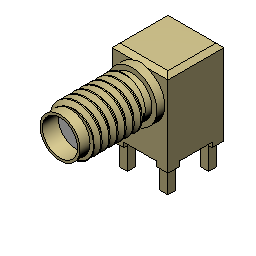
L-KLS1-SMA006 (Autodesk Fusion 360 design; units mm, degrees)
Autodesk Fusion 360 part; units mm, degrees
sketch "Sketch1" plane through (0, 0, 0) normal (0, 0, 1) x (1, 0, 0)
  circle A0 centre (0, 0) radius 0.65
  circle A1 centre (2.54, 2.54) radius 0.8
  circle A2 centre (-2.54, 2.54) radius 0.8
  circle A3 centre (-2.54, -2.54) radius 0.8
  circle A4 centre (2.54, -2.54) radius 0.8
  line L0 (3.04, 2.04) -> (2.04, 2.04)
  line L1 (2.04, 2.04) -> (2.04, 3.04)
  line L2 (2.04, 3.04) -> (3.04, 3.04)
  line L3 (3.04, 3.04) -> (3.04, 2.04)
  line L4 (3.04, 2.04) -> (2.04, 3.04) construction
  line L5 (2.04, 2.04) -> (3.04, 3.04) construction
  line L6 (-2.04, 2.04) -> (-3.04, 2.04)
  line L7 (-3.04, 2.04) -> (-3.04, 3.04)
  line L8 (-3.04, 3.04) -> (-2.04, 3.04)
  line L9 (-2.04, 3.04) -> (-2.04, 2.04)
  line L10 (-2.04, 2.04) -> (-3.04, 3.04) construction
  line L11 (-3.04, 2.04) -> (-2.04, 3.04) construction
  line L12 (-2.04, -2.04) -> (-3.04, -2.04)
  line L13 (-3.04, -2.04) -> (-3.04, -3.04)
  line L14 (-3.04, -3.04) -> (-2.04, -3.04)
  line L15 (-2.04, -3.04) -> (-2.04, -2.04)
  line L16 (-2.04, -2.04) -> (-3.04, -3.04) construction
  line L17 (-3.04, -2.04) -> (-2.04, -3.04) construction
  line L18 (3.04, -3.04) -> (2.04, -3.04)
  line L19 (2.04, -3.04) -> (2.04, -2.04)
  line L20 (2.04, -2.04) -> (3.04, -2.04)
  line L21 (3.04, -2.04) -> (3.04, -3.04)
  line L22 (3.04, -3.04) -> (2.04, -2.04) construction
  line L23 (2.04, -3.04) -> (3.04, -2.04) construction
  line L24 (3.5, 3.5) -> (3.5, -3.5)
  line L25 (-3.5, 3.5) -> (3.5, 3.5)
  line L26 (-3.5, -3.5) -> (-3.5, 3.5)
  line L27 (3.5, -3.5) -> (-3.5, -3.5)
  point P0 (2.54, 2.54)
  point P1 (2.54, 2.54)
  point P2 (-2.54, 2.54)
  point P3 (-2.54, -2.54)
  point P4 (2.54, -2.54)
  dimension "d1" = 1.3
  dimension "d2" = 1
  dimension "d3" = 1
  dimension "d4" = 1
  dimension "d5" = 1
  dimension "d6" = 1
  dimension "d7" = 1
  dimension "d8" = 1
  dimension "d9" = 1
  constraint coincident A0.centre origin
  constraint horizontal L0
  constraint perpendicular L0 L1
  constraint parallel L0 L2
  constraint parallel L1 L3
  constraint coincident L4 P1
  constraint coincident L5 P1
  constraint coincident P1 P0
  constraint horizontal L6
  constraint perpendicular L6 L7
  constraint parallel L6 L8
  constraint parallel L7 L9
  constraint coincident L10 P2
  constraint coincident L11 P2
  constraint coincident P2 A2.centre
  constraint horizontal L12
  constraint perpendicular L12 L13
  constraint parallel L12 L14
  constraint parallel L13 L15
  constraint coincident L16 P3
  constraint coincident L17 P3
  constraint coincident P3 A3.centre
  constraint horizontal L18
  constraint perpendicular L18 L19
  constraint parallel L18 L20
  constraint parallel L19 L21
  constraint coincident L22 P4
  constraint coincident L23 P4
  constraint coincident P4 A4.centre
  measures "d1" diameter of A0
  measures "d2" distance of L1.end L2.end
  measures "d3" distance of L0.end L1.end
  measures "d4" distance of L7.end L8.end
  measures "d5" distance of L6.end L7.end
  measures "d6" distance of L13.end L14.end
  measures "d7" distance of L12.end L13.end
  measures "d8" distance of L19.end L20.end
  measures "d9" distance of L18.end L19.end
extrude "Extrude1" add sketch "Sketch1" along normal blind 10.6 contours A0 | A1 | A2 | A3 | A4 | L0 L1 L2 L3 | L6 L7 L8 L9 | L12 L13 L14 L15 | L18 L19 L20 L21 | L24 L25 L26 L27
sketch "Sketch2" plane through (0, 0, 0) normal (0, 0, -1) x (1, 0, 0)
  line L0 (3.5, -3.5) -> (3.5, 3.5)
  line L1 (3.5, 3.5) -> (-3.5, 3.5)
  line L2 (-3.5, 3.5) -> (-3.5, -3.5)
  line L3 (-3.5, -3.5) -> (3.5, -3.5)
  circle A0 centre (2.54, 2.54) radius 0.8
  circle A1 centre (-2.54, 2.54) radius 0.8
  circle A2 centre (0, 0) radius 0.8
  circle A3 centre (-2.54, -2.54) radius 0.8
  circle A4 centre (2.54, -2.54) radius 0.8
  circle A5 centre (0, 0) radius 0.65
  line L4 (-2.04, 2.04) -> (-3.04, 2.04)
  line L5 (-3.04, 2.04) -> (-3.04, 3.04)
  line L6 (-3.04, 3.04) -> (-2.04, 3.04)
  line L7 (-2.04, 3.04) -> (-2.04, 2.04)
  line L8 (-2.04, 2.04) -> (-3.04, 3.04) construction
  line L9 (-3.04, 2.04) -> (-2.04, 3.04) construction
  line L10 (3.04, 2.04) -> (2.04, 2.04)
  line L11 (2.04, 2.04) -> (2.04, 3.04)
  line L12 (2.04, 3.04) -> (3.04, 3.04)
  line L13 (3.04, 3.04) -> (3.04, 2.04)
  line L14 (3.04, 2.04) -> (2.04, 3.04) construction
  line L15 (2.04, 2.04) -> (3.04, 3.04) construction
  line L16 (-2.04, -3.04) -> (-3.04, -3.04)
  line L17 (-3.04, -3.04) -> (-3.04, -2.04)
  line L18 (-3.04, -2.04) -> (-2.04, -2.04)
  line L19 (-2.04, -2.04) -> (-2.04, -3.04)
  line L20 (-2.04, -3.04) -> (-3.04, -2.04) construction
  line L21 (-3.04, -3.04) -> (-2.04, -2.04) construction
  line L22 (3.04, -3.04) -> (2.04, -3.04)
  line L23 (2.04, -3.04) -> (2.04, -2.04)
  line L24 (2.04, -2.04) -> (3.04, -2.04)
  line L25 (3.04, -2.04) -> (3.04, -3.04)
  line L26 (3.04, -3.04) -> (2.04, -2.04) construction
  line L27 (2.04, -3.04) -> (3.04, -2.04) construction
  point P0 (-2.54, 2.54)
  point P1 (2.54, 2.54)
  point P2 (-2.54, -2.54)
  point P3 (2.54, -2.54)
  dimension "d12" = 1.3
  dimension "d13" = 1
  dimension "d14" = 1
  dimension "d15" = 1
  dimension "d16" = 1
  dimension "d17" = 1
  dimension "d18" = 1
  dimension "d19" = 1
  dimension "d20" = 1
  constraint coincident A2.centre A5.centre
  constraint horizontal L4
  constraint perpendicular L4 L5
  constraint parallel L4 L6
  constraint parallel L5 L7
  constraint coincident L8 P0
  constraint coincident L9 P0
  constraint coincident P0 A1.centre
  constraint horizontal L10
  constraint perpendicular L10 L11
  constraint parallel L10 L12
  constraint parallel L11 L13
  constraint coincident L14 P1
  constraint coincident L15 P1
  constraint coincident P1 A0.centre
  constraint horizontal L16
  constraint perpendicular L16 L17
  constraint parallel L16 L18
  constraint parallel L17 L19
  constraint coincident L20 P2
  constraint coincident L21 P2
  constraint coincident P2 A3.centre
  constraint horizontal L22
  constraint perpendicular L22 L23
  constraint parallel L22 L24
  constraint parallel L23 L25
  constraint coincident L26 P3
  constraint coincident L27 P3
  constraint coincident P3 A4.centre
  measures "d12" diameter of A5
  measures "d13" distance of L5.end L6.end
  measures "d14" distance of L4.end L5.end
  measures "d15" distance of L11.end L12.end
  measures "d16" distance of L10.end L11.end
  measures "d17" distance of L17.end L18.end
  measures "d18" distance of L16.end L17.end
  measures "d19" distance of L23.end L24.end
  measures "d20" distance of L22.end L23.end
extrude "Extrude2" add sketch "Sketch2" along normal blind 2.8 contours A5 | L4 L5 L6 L7 | L10 L11 L12 L13 | L16 L17 L18 L19 | L22 L23 L24 L25
sketch "Sketch3" plane through (0, 0, 0) normal (0, 0, -1) x (1, 0, 0)
  circle A0 centre (0, 0) radius 0.65
  line L0 (3.04, 3.04) -> (3.04, 2.04)
  line L1 (3.04, 2.04) -> (2.04, 2.04)
  line L2 (2.04, 2.04) -> (2.04, 3.04)
  line L3 (2.04, 3.04) -> (3.04, 3.04)
  line L4 (-2.04, -2.04) -> (-2.04, -3.04)
  line L5 (-2.04, -3.04) -> (-3.04, -3.04)
  line L6 (-3.04, -3.04) -> (-3.04, -2.04)
  line L7 (-3.04, -2.04) -> (-2.04, -2.04)
  line L8 (-2.04, 3.04) -> (-2.04, 2.04)
  line L9 (-2.04, 2.04) -> (-3.04, 2.04)
  line L10 (-3.04, 2.04) -> (-3.04, 3.04)
  line L11 (-3.04, 3.04) -> (-2.04, 3.04)
  line L12 (3.04, -2.04) -> (3.04, -3.04)
  line L13 (3.04, -3.04) -> (2.04, -3.04)
  line L14 (2.04, -3.04) -> (2.04, -2.04)
  line L15 (2.04, -2.04) -> (3.04, -2.04)
  line L16 (3.5, -3.5) -> (3.5, 3.5)
  line L17 (3.5, 3.5) -> (-3.5, 3.5)
  line L18 (-3.5, 3.5) -> (-3.5, -3.5)
  line L19 (-3.5, -3.5) -> (3.5, -3.5)
  line L20 (3.5, -2.04) -> (-3.5, -2.04)
  line L21 (-3.5, -2.04) -> (-3.5, 2.04)
  line L22 (-3.5, 2.04) -> (3.5, 2.04)
  line L23 (3.5, 2.04) -> (3.5, -2.04)
  line L24 (3.5, -2.04) -> (-3.5, 2.04) construction
  line L25 (-3.5, -2.04) -> (3.5, 2.04) construction
  line L26 (2.04, -3.5) -> (-2.04, -3.5)
  line L27 (-2.04, -3.5) -> (-2.04, 3.5)
  line L28 (-2.04, 3.5) -> (2.04, 3.5)
  line L29 (2.04, 3.5) -> (2.04, -3.5)
  line L30 (2.04, -3.5) -> (-2.04, 3.5) construction
  line L31 (-2.04, -3.5) -> (2.04, 3.5) construction
  constraint horizontal L20
  constraint perpendicular L20 L21
  constraint parallel L20 L22
  constraint parallel L21 L23
  constraint coincident L24 A0.centre
  constraint coincident L25 A0.centre
  constraint coincident L16 L20.start
  constraint coincident A0.centre origin
  constraint horizontal L26
  constraint perpendicular L26 L27
  constraint parallel L26 L28
  constraint parallel L27 L29
  constraint coincident L30 A0.centre
  constraint coincident L31 A0.centre
  constraint coincident L19 L26.start
extrude "Extrude3" cut sketch "Sketch3" against normal blind 0.6 contours L1 L15 L16 L20 L22 L23 L29 | L2 L8 L17 L22 L27 L28 L29 | L20 L22 L27 L29 | L7 L9 L18 L20 L21 L22 L27 | L4 L14 L19 L20 L26 L27 L29
sketch "Sketch4" plane through (0, -3.5, 0) normal (0, -1, 0) x (1, 0, 0)
  line L0 (-2.04, 0) -> (-2.04, 0.6)
  line L1 (-2.04, 0.6) -> (2.04, 0.6)
  line L2 (2.04, 0.6) -> (2.04, 0)
  line L3 (2.04, 0) -> (3.5, 0)
  line L4 (3.5, 0) -> (3.5, 10.6)
  line L5 (3.5, 10.6) -> (-3.5, 10.6)
  line L6 (-3.5, 10.6) -> (-3.5, 0)
  line L7 (-3.5, 0) -> (-2.04, 0)
  line L8 (0, 10.6) -> (0, 3.6) construction
  circle A0 centre (0, 7.1) radius 3.1
  dimension "d25" = 7
  dimension "d26" = 6.2
  constraint midpoint L5 L8.start
  constraint perpendicular L5 L8
  constraint midpoint L8 A0.centre
  measures "d25" distance of L8.start L8.end
  measures "d26" diameter of A0
extrude "Extrude4" add sketch "Sketch4" along normal blind 1 contours A0
sketch "Sketch5" plane through (0, -4.5, 0) normal (0, -1, 0) x (1, 0, 0)
  circle A0 centre (0, 7.1) radius 3.1
  circle A1 centre (0, 7.1) radius 2.5
  dimension "d29" = 5
  constraint concentric A0 A1
  measures "d29" diameter of A1
extrude "Extrude5" add sketch "Sketch5" along normal blind 1 contours A1
sketch "Sketch6" plane through (0, -5.5, 0) normal (0, -1, 0) x (1, 0, 0)
  circle A0 centre (0, 7.1) radius 2.5
  circle A1 centre (0, 7.1) radius 3.1
  dimension "d32" = 6.2
  constraint concentric A0 A1
  measures "d32" diameter of A1
extrude "Extrude6" add sketch "Sketch6" along normal blind 6.75 contours A0 | A1
sketch "Sketch7" plane through (0, -12.25, 0) normal (0, -1, 0) x (1, 0, 0)
  circle A0 centre (0, 7.1) radius 3.1
  circle A1 centre (0, 7.1) radius 2.5
  dimension "d35" = 5
  constraint concentric A0 A1
  measures "d35" diameter of A1
extrude "Extrude7" add sketch "Sketch7" along normal blind 1.25 contours A1
thread "Thread1" "ISO Metric profile 6.0 M6x1 6g" major diameter 5.884 minor diameter 4.7435 pitch 1 angle 60 modelled right hand crest width 0.1444 on face at (3.0961, -10, 6.9455) crest through (2.942, -5.25, 7.1)
sketch "Sketch8" plane through (0, -13.5, 0) normal (0, -1, 0) x (1, 0, 0)
  circle A0 centre (0, 7.1) radius 2.5
  circle A1 centre (0, 7.1) radius 2.2
  dimension "d38" = 4.4
  constraint concentric A0 A1
  measures "d38" diameter of A1
extrude "Extrude8" cut sketch "Sketch8" against normal blind 2 contours A1
sketch "Sketch9" plane through (0, -11.5, 0) normal (0, -1, 0) x (1, 0, 0)
  circle A0 centre (0, 7.1) radius 2.2
  circle A1 centre (0, 7.1) radius 0.25
  circle A2 centre (0, 7.1) radius 0.3
  dimension "d41" = 0.5
  dimension "d42" = 0.6
  constraint concentric A0 A1
  constraint concentric A0 A2
  measures "d41" diameter of A1
  measures "d42" diameter of A2
extrude "Extrude9" cut sketch "Sketch9" against normal blind 3 contours A1
extrude "Extrude10" add sketch "Sketch9" along normal blind 0.05 contours A2
chamfer "Chamfer1" distance 0.5 angle 45 4 edges at (-3.5, 0, 10.6) (0, -3.5, 10.6) (3.5, 0, 10.6) (0, 3.5, 10.6)
sketch "Sketch11" plane through (0, -11.5, 7.1) normal (0, -1, 0) x (1, 0, 0)
  circle A0 centre (0, 0) radius 2.1
  dimension "d51" = 4.2
  constraint coincident A0.centre origin
  measures "d51" diameter of A0
sketch "Sketch12" plane through (0, 0, 0.6) normal (0, 0, -1) x (1, 0, 0)
  circle A0 centre (0, 0) radius 0.65
  line L0 (2.04, 3.5) -> (-2.04, 3.5)
  line L1 (-2.04, 3.5) -> (-2.04, 2.04)
  line L2 (-2.04, 2.04) -> (-3.5, 2.04)
  line L3 (-3.5, 2.04) -> (-3.5, -2.04)
  line L4 (-3.5, -2.04) -> (-2.04, -2.04)
  line L5 (-2.04, -2.04) -> (-2.04, -3.5)
  line L6 (-2.04, -3.5) -> (2.04, -3.5)
  line L7 (2.04, -3.5) -> (2.04, -2.04)
  line L8 (2.04, -2.04) -> (3.5, -2.04)
  line L9 (3.5, -2.04) -> (3.5, 2.04)
  line L10 (3.5, 2.04) -> (2.04, 2.04)
  line L11 (2.04, 2.04) -> (2.04, 3.5)
  circle A1 centre (0, 0) radius 2
  dimension "d56" = 4
  constraint coincident A0.centre A1.centre
  measures "d56" diameter of A1
extrude "Extrude14" cut sketch "Sketch12" against normal blind 0.5 contours A1
equation "d10 = 13.4 mm - 2.8 mm"
